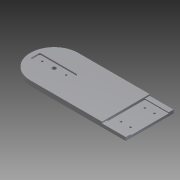
# Autodesk Inventor part: plancha base
Saved by Autodesk Inventor 2011 (Build 150239000, 239)
## iProperties
Created: 2010-08-08
Part Number: plancha base
Document SubType Name: Modeling
Designer: lucio
Density: 1 g/cm^3
Author: lucio
Autodesk Inventor part; units mm, degrees
ref_plane "YZ Plane" through (0, 0, 0) normal (1, 0, 0) x (0, 1, 0)
ref_plane "XZ Plane" through (0, 0, 0) normal (0, 1, 0) x (-1, 0, 0)
ref_plane "XY Plane" through (0, 0, 0) normal (0, 0, 1) x (1, 0, 0)
sketch "Sketch1" plane through (0, 0, 0) normal (0, 0, 1) x (1, 0, 0)
  line L0 (232.6946, -90.5389) -> (32.6946, -90.5389)
  line L1 (-17.3054, -40.5389) -> (-17.3054, -40.5389)
  line L2 (32.6946, 9.4611) -> (232.6946, 9.4611)
  line L3 (232.6946, 9.4611) -> (232.6946, -90.5389)
  circle A0 centre (32.6946, -40.5389) radius 4
  arc A1 (-17.3054, -40.5389) -> (32.6946, -90.5389) centre (32.6946, -40.5389) ccw
  arc A2 (32.6946, 9.4611) -> (-17.3054, -40.5389) centre (32.6946, -40.5389) ccw
  point P0 (0, 0)
  point P1 (-17.3054, 9.4611)
  point P2 (-17.3054, -90.5389)
  dimension "d0" = 250
  dimension "d1" = 100
  dimension "d2" = 8
  dimension "d3" = 50
  dimension "d4" = 50
  dimension "d5" = 50
  constraints: 8 end point, 4 point on circle, 4 point on line, 4 tangent, 3 centre point, 2 parallel, 1 concentric, 1 horizontal, 1 perpendicular
  measures "d0" distance of point (-17.305, 9.461) L2.end
  measures "d1" distance of point (-17.305, -90.539) point (-17.305, 9.461)
  measures "d2" diameter of A0
  measures "d3" distance from line of L1 A0.centre
  measures "d4" distance from line of L2 A0.centre
  measures "d5" radius of A1
extrude "Extrusion1" add sketch "Sketch1" along normal blind 10
sketch "Sketch2" plane through (0, 0, 10) normal (0, 0, 1) x (1, 0, 0)
  line L0 (32.6946, 9.4611) -> (232.6946, 9.4611) projected
  line L1 (232.6946, -90.5389) -> (182.6946, -90.5389)
  line L2 (182.6946, -90.5389) -> (182.6946, 9.4611)
  line L3 (182.6946, 9.4611) -> (232.6946, 9.4611)
  line L4 (232.6946, 9.4611) -> (232.6946, -90.5389)
  point P0 (0, 0)
  dimension "d8" = 50
  constraints: 8 end point, 2 parallel, 1 horizontal, 1 perpendicular, 1 point on line
  measures "d8" distance between parallel lines of L4 L2
extrude "Extrusion2" cut sketch "Sketch2" against normal blind 5
sketch "Sketch3" plane through (0, 0, 5) normal (0, 0, 1) x (1, 0, 0)
  line L0 (182.6946, 9.4611) -> (232.6946, 9.4611) projected
  line L1 (182.6946, 9.4611) -> (182.6946, -90.5389) projected
  line L2 (232.6946, -90.5389) -> (182.6946, -90.5389) projected
  line L3 (232.6946, 9.4611) -> (232.6946, -90.5389) projected
  point P0 (0, 0)
  point P1 (197.6946, -65.5389)
  point P2 (197.6946, -15.5389)
  point P3 (217.6946, -15.5389)
  point P4 (217.6946, -65.5389)
  dimension "d11" = 15
  dimension "d12" = 25
  dimension "d13" = 25
  dimension "d14" = 15
  constraints: 2 horizontal alignment, 2 vertical alignment
  measures "d11" distance from line of L1 point (197.695, -65.539)
  measures "d12" distance from line of L2 point (197.695, -65.539)
  measures "d13" distance from line of L0 point (217.695, -15.539)
  measures "d14" distance from line of L3 point (217.695, -15.539)
hole "Hole1" at (197.6946, -65.5389, 5) at (197.6946, -15.5389, 5) at (217.6946, -15.5389, 5) at (217.6946, -65.5389, 5) direction (0, 0, -1) diameter 4 end through all
sketch "Sketch4" plane through (0, 0, 10) normal (0, 0, 1) x (1, 0, 0)
  arc A0 (32.6946, 9.4611) -> (32.6946, -90.5389) centre (32.6946, -40.5389) ccw projected
  point P0 (0, 0)
  point P1 (7.6946, -40.5389)
  point P2 (57.6946, -40.5389)
  dimension "d22" = 25
  dimension "d23" = 25
  constraints: 2 horizontal alignment
  measures "d22" distance of A0.centre point (7.695, -40.539)
  measures "d23" distance of point (57.695, -40.539) A0.centre
hole "Hole2" at (7.6946, -40.5389, 10) at (57.6946, -40.5389, 10) direction (0, 0, -1) diameter 4 end through all
sketch "Sketch5" plane through (0, 0, 10) normal (0, 0, 1) x (1, 0, 0)
  circle A0 centre (57.6946, -40.5389) radius 2 projected
  circle A1 centre (7.6946, -40.5389) radius 2 projected
  arc A2 (32.6946, 9.4611) -> (32.6946, -90.5389) centre (32.6946, -40.5389) ccw projected
  circle A3 centre (32.6946, -40.5389) radius 4 projected
  line L0 (72.6946, -50.5389) -> (-7.3054, -50.5389)
  line L1 (-7.3054, -50.5389) -> (-7.3054, -30.5389)
  line L2 (-7.3054, -30.5389) -> (72.6946, -30.5389)
  line L3 (72.6946, -30.5389) -> (72.6946, -50.5389)
  point P0 (0, 0)
  dimension "d35" = 80
  dimension "d36" = 20
  dimension "d37" = 40
  dimension "d38" = 10
  constraints: 8 end point, 2 parallel, 1 horizontal, 1 perpendicular
  measures "d35" distance of L1.end L2.end
  measures "d36" distance of L0.end L1.end
  measures "d37" distance from line of A2.centre L1
  measures "d38" distance from line of L0 A1.centre
extrude "Extrusion3" cut sketch "Sketch5" against normal blind 3
sketch "Sketch6" plane through (0, 0, 5) normal (0, 0, 1) x (1, 0, 0)
  line L0 (232.6946, 9.4611) -> (232.6946, -90.5389) projected
  line L1 (182.6946, -90.5389) -> (232.6946, -90.5389)
  line L2 (232.6946, -90.5389) -> (232.6946, -80.5389)
  line L3 (232.6946, -80.5389) -> (182.6946, -80.5389)
  line L4 (182.6946, -80.5389) -> (182.6946, -90.5389)
  line L5 (182.6946, 9.4611) -> (232.6946, 9.4611)
  line L6 (232.6946, 9.4611) -> (232.6946, -0.5389)
  line L7 (232.6946, -0.5389) -> (182.6946, -0.5389)
  line L8 (182.6946, -0.5389) -> (182.6946, 9.4611)
  point P0 (0, 0)
  dimension "d41" = 10
  dimension "d42" = 10
  constraints: 16 end point, 4 parallel, 2 horizontal, 2 perpendicular, 2 point on line
  measures "d41" distance of L1.end L2.end
  measures "d42" distance between parallel lines of L7 L5
extrude "Extrusion4" add sketch "Sketch6" along normal blind 2
fillet "Fillet1" radius 2 2 edges at (182.6946, -0.5389, 6) (182.6946, -80.5389, 6)
fillet "Fillet2" radius 3 4 edges at (-7.3054, -30.5389, 8.5) (-7.3054, -50.5389, 8.5) (72.6946, -30.5389, 8.5) (72.6946, -50.5389, 8.5)
equation "\"d4\" = 0.5 * d1"
equation "\"d23\" = d22"
equation "\"d37\" = 0.5 * d35"
equation "\"d38\" = 0.5 * d36"
body "Solid1"
